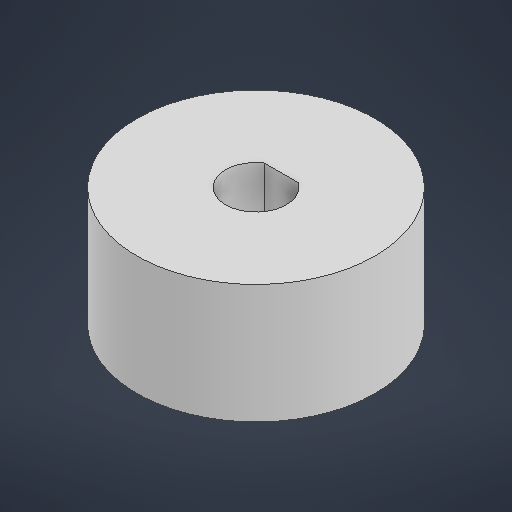
# Autodesk Inventor part: steppermotorcap
Saved by Autodesk Inventor 2027.1 (Build 311267000, 267)
## iProperties
Created: 2026-10-02
Part Number: steppermotorcap
Material: Generic
Document SubType Name: Modeling
Designer: HP
Density: 1 g/cm^3
Appearance: Default
Author: HP
Autodesk Inventor part; units mm, degrees
ref_plane "YZ Plane" through (0, 0, 0) normal (1, 0, 0) x (0, 1, 0)
ref_plane "XZ Plane" through (0, 0, 0) normal (0, 1, 0) x (-1, 0, 0)
ref_plane "XY Plane" through (0, 0, 0) normal (0, 0, 1) x (1, 0, 0)
sketch "Sketch1" plane through (0, 0, 0) normal (0, 1, 0) x (-1, 0, 0)
  circle A0 centre (5.406, 6.5732) radius 10
  point P0 (0, 0)
  dimension "d0" = 20
  constraints: 1 centre point
  measures "d0" diameter of A0
extrude "Extrusion1" add sketch "Sketch1" along normal blind 10
sketch "Sketch4" plane through (-5.406, 10, 6.5732) normal (0, 1, 0) x (1, 0, 0)
  circle A0 centre (0, 0) radius 2.5527
  circle A1 centre (0, 0) radius 10 projected
  line L0 (-1.4351, 2.1111) -> (1.4351, 2.1111)
  point P0 (5.406, 6.5732)
  dimension "d10" = 5.1054
  dimension "d11" = 2.8702
  constraints: 2 end point, 2 point on circle, 1 centre point, 1 concentric, 1 horizontal
  measures "d10" diameter of A0
  measures "d11" distance of L0.start L0.end
extrude "Extrusion3" cut sketch "Sketch4" against normal blind 50 contours A0 L0 picked at (0.1004, 0.5624)
body "Solid1"
